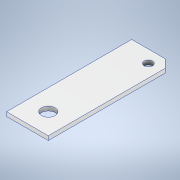
# Autodesk Inventor part: spring cover
Saved by Autodesk Inventor 2022 (Build 260153000, 153)
## iProperties
Created: 2022-02-18
Part Number: spring cover
Material: Aluminum 6061
Document SubType Name: Modeling
Designer: Bowen
Density: 2.7 g/cm^3
Appearance: Aluminum - Flat
Author: Bowen
Autodesk Inventor part; units mm, degrees
ref_plane "YZ Plane" through (0, 0, 0) normal (1, 0, 0) x (0, 1, 0)
ref_plane "XZ Plane" through (0, 0, 0) normal (0, 1, 0) x (-1, 0, 0)
ref_plane "XY Plane" through (0, 0, 0) normal (0, 0, 1) x (1, 0, 0)
sketch "Sketch1" plane through (0, 0, 0) normal (0, 1, 0) x (-1, 0, 0)
  line L0 (5, 15) -> (-5, 15)
  line L1 (-5, 15) -> (-5, -15)
  line L2 (-5, -15) -> (5, -15)
  line L3 (5, -15) -> (5, 15)
  point P0 (0, 0)
  point P1 (5, 0)
  point P2 (0, -15)
  dimension "d0" = 30
  dimension "d1" = 10
  constraints: 8 end point, 2 midpoint, 2 parallel, 1 horizontal, 1 horizontal alignment, 1 perpendicular, 1 vertical alignment
  measures "d0" distance of L2.end L0.start
  measures "d1" distance of L1.end L2.end
extrude "Extrusion1" add sketch "Sketch1" along normal blind 1
sketch "Sketch2" plane through (0, 1, 0) normal (0, 1, 0) x (1, 0, 0)
  line L0 (-5, -15) -> (5, -15) projected
  point P0 (0, 0)
  point P1 (0, -10)
  dimension "d4" = 5
  constraints: 1 vertical alignment
  measures "d4" distance from line of L0 point (0, -10)
hole "Hole1" at (0, 1, 10) direction (0, -1, 0) diameter 3.264 depth 4 clearance for "Flat Head Machine Screw (82)" size "#4" standard "Ansi Unified Screw Threads"
chamfer "Chamfer1" distance 2 angle 45 1 edges at (5, 0.5, -15)
sketch "Sketch3" plane through (0, 1, 0) normal (0, 1, 0) x (1, 0, 0)
  line L0 (5, -15) -> (5, 13) projected
  line L1 (3, 15) -> (-5, 15) projected
  point P0 (0, 0)
  point P1 (2, 12)
  dimension "d15" = 3
  dimension "d16" = 3
  measures "d15" distance from line of L0 point (2, 12)
  measures "d16" distance from line of L1 point (2, 12)
hole "Hole2" at (2, 1, -12) direction (0, -1, 0) diameter 2 end through all
body "Solid1"
